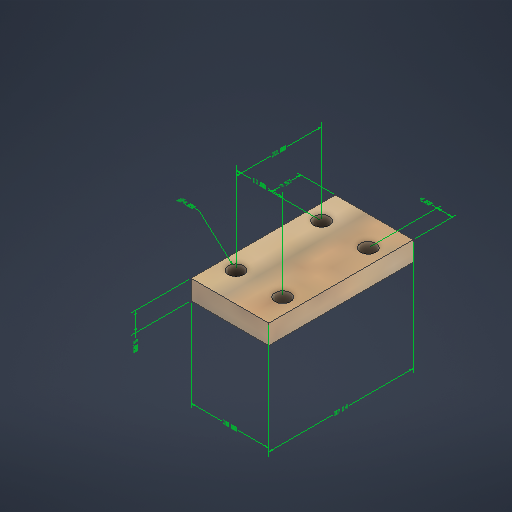
# Autodesk Inventor part: Sujetador
Saved by Autodesk Inventor 2026.2 (Build 302298000, 298)
## iProperties
Created: 2026-02-22
Part Number: Sujetador
Material: Genérico
Document SubType Name: Sheet Metal
Designer: yahir
Density: 1 g/cm^3
Sheet Metal Rule: Por defecto_mm
Appearance: Valor por defecto
Author: yahir
Autodesk Inventor part; units mm, degrees
ref_plane "YZ Plane" through (0, 0, 0) normal (1, 0, 0) x (0, 1, 0)
ref_plane "XZ Plane" through (0, 0, 0) normal (0, 1, 0) x (-1, 0, 0)
ref_plane "XY Plane" through (0, 0, 0) normal (0, 0, 1) x (1, 0, 0)
sketch "Boceto1" plane through (0, 0, 0) normal (0, 1, 0) x (-1, 0, 0)
  line L0 (4, 5) -> (4, 18.57)
  line L1 (4, 18.57) -> (-16, 18.57)
  line L2 (-16, 18.57) -> (-16, -18.57)
  line L3 (-16, -18.57) -> (4, -18.57)
  line L4 (4, -18.57) -> (4, -5)
  line L5 (0, -5) -> (0, -11)
  line L6 (0, 5) -> (0, 11)
  line L7 (0, -11) -> (-12, -11)
  line L8 (0, 11) -> (-12, 11)
  circle A0 centre (0, 11) radius 2
  circle A1 centre (0, -11) radius 2
  circle A2 centre (-12, -11) radius 2
  circle A3 centre (-12, 11) radius 2
  line L9 (4, -5) -> (4, 5)
  point P0 (0, 0)
  dimension "d0" = 5
  dimension "d1" = 4
  dimension "d2" = 13.57
  dimension "d3" = 20
  dimension "d4" = 37.14
  dimension "d5" = 20
  dimension "d6" = 13.57
  dimension "d7" = 4
  dimension "d8" = 6
  dimension "d9" = 6
  dimension "d11" = 12
  dimension "d12" = 12
  dimension "d13" = 4
  dimension "d14" = 4
  dimension "d15" = 4
  dimension "d16" = 4
  constraints: 20 end point, 4 centre point, 4 coincident, 3 horizontal, 3 perpendicular, 3 vertical
  measures "d0" distance of point (0, 0) L6.start
  measures "d1" distance of L6.start L0.start
  measures "d2" distance of L0.start L0.end
  measures "d3" distance of L0.end L1.end
  measures "d4" distance of L1.end L2.end
  measures "d5" distance of L2.end L3.end
  measures "d6" distance of L3.end L4.end
  measures "d7" distance of L4.end L5.start
  measures "d8" distance of L5.start L5.end
  measures "d9" distance of L6.start L6.end
  measures "d11" distance of L5.end L7.end
  measures "d12" distance of L6.end L8.end
  measures "d13" diameter of A0
  measures "d14" diameter of A1
  measures "d15" diameter of A2
  measures "d16" diameter of A3
extrude "Extrusión1" add sketch "Boceto1" along normal blind 5
equation "\"Radio_pliegue\" = Grosor"
equation "\"Anchura_desahogo_plegado\" = Grosor"
equation "\"Profundidad_desahogo_plegado\" = 0.5 * Grosor"
equation "\"Tamaño_destalonado\" = 4 * Grosor"
equation "\"Remanente_mínimo\" = 2 * Grosor"
equation "\"Radiodetransición\" = Radio_pliegue"
equation "\"Tamaño_de_radio_de_Jacobi\" = Radio_pliegue"
equation "\"TamañoSeparación\" = Grosor"
equation "\"Grosor\" = 0.5"
